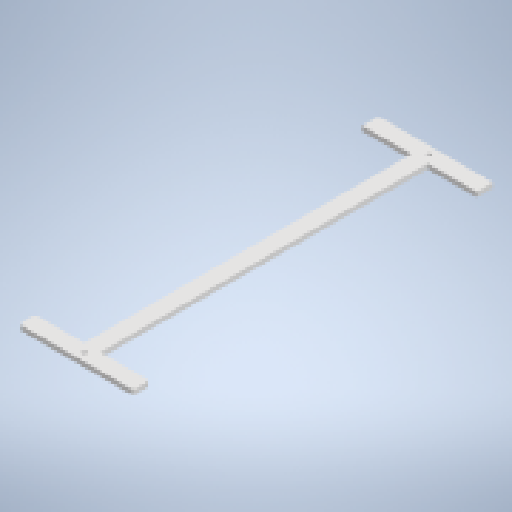
# Autodesk Inventor part: Tensor
Saved by Autodesk Inventor 2024 (Build 280153000, 153)
## iProperties
Created: 2025-02-23
Part Number: Tensor
Material: Genérico
Document SubType Name: Modeling
Designer: sergi
Density: 1 g/cm^3
Appearance: Valor por defecto
Author: sergi
Autodesk Inventor part; units mm, degrees
ref_plane "YZ Plane" through (0, 0, 0) normal (1, 0, 0) x (0, 1, 0)
ref_plane "XZ Plane" through (0, 0, 0) normal (0, 1, 0) x (-1, 0, 0)
ref_plane "XY Plane" through (0, 0, 0) normal (0, 0, 1) x (1, 0, 0)
sketch "Boceto1" plane through (0, 0, 0) normal (0, 1, 0) x (-1, 0, 0)
  line L0 (-2, 110) -> (2, 110)
  line L1 (5, 107) -> (5, -107)
  line L2 (2, -110) -> (-2, -110)
  line L3 (-5, -107) -> (-5, 107)
  line L4 (-5, 110) -> (5, -110) construction
  line L5 (5, 110) -> (-5, -110) construction
  arc A0 (5, 107) -> (2, 110) centre (2, 107) ccw
  arc A1 (-2, 110) -> (-5, 107) centre (-2, 107) ccw
  arc A2 (-5, -107) -> (-2, -110) centre (-2, -107) ccw
  arc A3 (2, -110) -> (5, -107) centre (2, -107) ccw
  line L6 (-2, 110) -> (-5, 110)
  line L7 (-5, 110) -> (-35, 110)
  line L8 (-35, 110) -> (-35, 100)
  line L9 (-35, 100) -> (-5, 100)
  line L10 (-2, 110) -> (5, 110)
  line L11 (5, 110) -> (35, 110)
  line L12 (35, 110) -> (35, 100)
  line L13 (35, 100) -> (-5, 100)
  line L14 (35, -100) -> (35, -110)
  line L15 (35, -110) -> (-35, -110)
  line L16 (-35, -110) -> (-35, -100)
  line L17 (-35, -100) -> (35, -100)
  line L18 (35, -100) -> (35, -110)
  point P0 (0, 0)
  point P1 (2, 110)
  point P2 (5, 100)
  point P3 (-2, -110)
  point P4 (-5, -100)
  point P5 (5, -100)
  dimension "d0" = 10
  dimension "d1" = 220
  dimension "d2" = 3
  dimension "d16" = 3
  dimension "d17" = 30
  dimension "d18" = 10
  dimension "d19" = 7
  dimension "d20" = 30
  dimension "d21" = 10
  dimension "d36" = 70
  constraints: 38 end point, 13 point on line, 9 tangent, 8 point on circle, 5 perpendicular, 4 centre point, 4 parallel, 3 equal radius, 3 horizontal, 2 midpoint, 1 collinear
  measures "d0" distance of L4.end L5.end
  measures "d1" distance of L5.start L4.end
  measures "d2" radius of A0
  measures "d16" distance of L0.start L4.start
  measures "d17" distance of L4.start L7.end
  measures "d18" distance of L7.end L8.end
  measures "d19" distance of L0.start L5.start
  measures "d20" distance of L5.start L11.end
  measures "d21" distance of L11.end L12.end
  measures "d36" distance of L16.end L17.end
extrude "Extrusión1" add sketch "Boceto1" along normal blind 3
sketch "Boceto3" plane through (0, 3, 0) normal (0, 1, 0) x (1, 0, 0)
  line L0 (-35, -110) -> (35, -110) projected
  line L1 (5, -100) -> (5, 100) projected
  line L2 (35, 110) -> (-35, 110) projected
  line L3 (-5, 100) -> (-5, -100) projected
  point P0 (0, 0)
  point P1 (0, -105)
  point P2 (5, 107)
  point P3 (0.8679, 105)
  dimension "d23" = 5
  dimension "d24" = 5
  dimension "d37" = 5
  dimension "d38" = 5.8679
  measures "d23" distance from line of L0 point (0, -105)
  measures "d24" distance from line of L1 point (0, -105)
  measures "d37" distance from line of L2 point (0.868, 105)
  measures "d38" distance from line of L3 point (0.868, 105)
hole "Agujero2" at (0, 3, 105) at (0.8679, 3, -105) direction (0, -1, 0) diameter 3 end through all
fillet "Empalme1" radius 2 5 edges at (35, 1.5, 100) (35, 1.5, 110) (-35, 1.5, 110) (-35, 1.5, 100) (-35, 1.5, -110)
